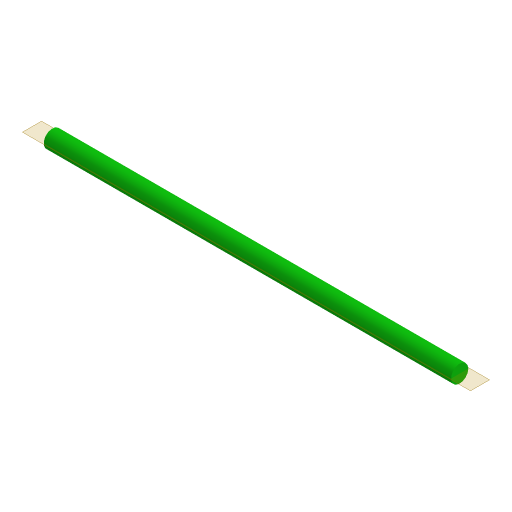
# Autodesk Inventor part: Шпилька
Saved by Autodesk Inventor 2023.2 (Build 272271030, 271C)
## iProperties
Created: 2024-02-21
Part Number: Шпилька
Material: Типовые
Document SubType Name: Modeling
Designer: I9232
Density: 1 g/cm^3
Appearance: По умолчанию
Author: I9232
Autodesk Inventor part; units mm, degrees
ref_plane "YZ Plane" through (0, 0, 0) normal (1, 0, 0) x (0, 1, 0)
ref_plane "XY Plane" through (0, 0, 0) normal (0, 0, 1) x (1, 0, 0)
sketch "Эскиз1" plane through (0, 0, 0) normal (0, 1, 0) x (-1, 0, 0)
  line L0 (94, 0) -> (94, -4)
  line L1 (94, -4) -> (0, -4)
  line L2 (0, -4) -> (0, 0) construction
  line L3 (-94, 0) -> (-94, -4)
  line L4 (-94, -4) -> (0, -4)
  line L5 (1.8444, 0) -> (-1.3044, 0) construction
  line L6 (94, 0) -> (-94, 0)
  dimension "d0" = 4
  dimension "d1" = 94
  constraints: 14 end point, 2 horizontal, 2 symmetric about line, 1 collinear, 1 midpoint, 1 parallel
  measures "d0" distance of L0.start L0.end
  measures "d1" distance of L0.end L1.end
revolve "Вращение1" add sketch "Эскиз1" angle 360 about axis through (-1.8444, 0, 0) along (1, 0, 0)
